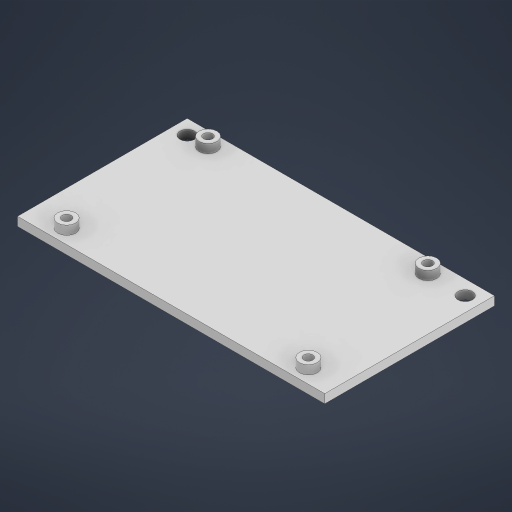
# Autodesk Inventor part: placa_arduino
Saved by Autodesk Inventor 2023 (Build 270158000, 158)
## iProperties
Created: 2022-08-23
Part Number: placa_arduino
Material: Generic
Document SubType Name: Modeling
Designer: marat
Density: 1 g/cm^3
Appearance: Default
Author: marat
Autodesk Inventor part; units mm, degrees
ref_plane "YZ Plane" through (0, 0, 0) normal (1, 0, 0) x (0, 1, 0)
ref_plane "XZ Plane" through (0, 0, 0) normal (0, 1, 0) x (-1, 0, 0)
ref_plane "XY Plane" through (0, 0, 0) normal (0, 0, 1) x (1, 0, 0)
sketch "Sketch1" plane through (0, 0, 0) normal (0, 1, 0) x (-1, 0, 0)
  line L0 (52.5, 29) -> (-52.5, 29)
  line L1 (-52.5, 29) -> (-52.5, -29)
  line L2 (-52.5, -29) -> (52.5, -29)
  line L3 (52.5, -29) -> (52.5, 29)
  line L4 (52.5, 29) -> (-52.5, -29) construction
  line L5 (-52.5, 29) -> (52.5, -29) construction
  point P0 (0, 0)
  dimension "d0" = 105
  dimension "d1" = 58
  constraints: 12 end point, 2 midpoint, 2 parallel, 1 horizontal, 1 perpendicular
  measures "d0" distance of L2.end L1.end
  measures "d1" distance of L1.end L0.end
extrude "Extrusion1" add sketch "Sketch1" along normal blind 3
sketch "Sketch2" plane through (0, 3, 0) normal (0, 1, 0) x (1, 0, 0)
  circle A0 centre (41.9878, -24.0965) radius 1.562
  circle A1 centre (41.9878, -24.0965) radius 3.062
  circle A2 centre (-40.6382, -24.0965) radius 1.562
  circle A3 centre (-40.6382, -24.0965) radius 3.062
  circle A4 centre (-40.6382, 24.2395) radius 1.562
  circle A5 centre (-40.6382, 24.2395) radius 3.062
  circle A6 centre (34.4948, 24.2395) radius 1.562
  circle A7 centre (34.4948, 24.2395) radius 3.062
  point P0 (0, 0)
  dimension "d4" = 3.124
  dimension "d5" = 1.5
  dimension "d6" = 3.124
  dimension "d7" = 1.5
  dimension "d8" = 82.626
  dimension "d9" = 3.124
  dimension "d10" = 1.5
  dimension "d11" = 48.336
  dimension "d12" = 3.124
  dimension "d13" = 1.5
  dimension "d14" = 75.133
  dimension "d15" = 0
  dimension "d16" = 0
  constraints: 8 centre point
  measures "d4" diameter of A0
  measures "d5" radial gap between concentric circles of A0 A1
  measures "d6" diameter of A2
  measures "d7" radial gap between concentric circles of A2 A3
  measures "d8" distance of A0.centre A2.centre
  measures "d9" diameter of A4
  measures "d10" radial gap between concentric circles of A4 A5
  measures "d11" distance of A4.centre A2.centre
  measures "d12" diameter of A6
  measures "d13" radial gap between concentric circles of A6 A7
  measures "d14" distance of A6.centre A4.centre
  measures "d15" vertical distance of A0.centre A2.centre
  measures "d16" horizontal distance of A4.centre A2.centre
extrude "Extrusion2" add sketch "Sketch2" along normal blind 3
sketch "Sketch3" plane through (0, 3, 0) normal (0, 1, 0) x (1, 0, 0)
  circle A0 centre (47.5, 24) radius 2.5
  line L0 (52.5, 29) -> (-52.5, 29) projected
  line L1 (52.5, -29) -> (52.5, 29) projected
  circle A1 centre (-47.5, 24) radius 2.5
  line L2 (-52.5, 29) -> (-52.5, -29) projected
  point P0 (0, 0)
  dimension "d19" = 5
  dimension "d20" = 5
  dimension "d21" = 5
  dimension "d22" = 5
  dimension "d23" = 5
  dimension "d24" = 5
  constraints: 2 centre point
  measures "d19" diameter of A0
  measures "d20" distance from line of L0 A0.centre
  measures "d21" distance from line of L1 A0.centre
  measures "d22" diameter of A1
  measures "d23" distance from line of L2 A1.centre
  measures "d24" distance from line of L0 A1.centre
extrude "Extrusion3" cut sketch "Sketch3" against normal through all
body "Solid1"
